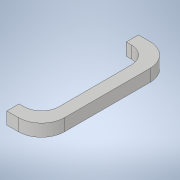
# Autodesk Inventor part: acc door handle
Saved by Autodesk Inventor 2020 (Build 240168000, 168)
## iProperties
Created: 2019-03-08
Part Number: acc door handle
Material: Generic
Document SubType Name: Modeling
Designer: aonih
Density: 1 g/cm^3
Appearance: Default
Author: aonih
Autodesk Inventor part; units mm, degrees
ref_plane "YZ Plane" through (0, 0, 0) normal (1, 0, 0) x (0, 1, 0)
ref_plane "XZ Plane" through (0, 0, 0) normal (0, 1, 0) x (-1, 0, 0)
ref_plane "XY Plane" through (0, 0, 0) normal (0, 0, 1) x (1, 0, 0)
sketch "Sketch1" plane through (0, 0, 0) normal (0, 1, 0) x (-1, 0, 0)
  line L0 (15, 57) -> (-15, 57)
  line L1 (-15, 57) -> (-15, -57)
  line L2 (-15, -57) -> (15, -57)
  line L3 (15, -57) -> (15, 57)
  line L4 (0, 57) -> (0, -57) construction
  line L5 (15, 0) -> (-15, 0) construction
  line L6 (15, 46.3934) -> (10.6066, 46.3934)
  line L7 (-4.3934, 31.3934) -> (-4.3934, -31.3934)
  line L8 (10.6066, -46.3934) -> (15, -46.3934)
  line L9 (15, -46.3934) -> (15, 46.3934)
  arc A0 (10.6066, 46.3934) -> (-4.3934, 31.3934) centre (10.6066, 31.3934) ccw
  arc A1 (-4.3934, -31.3934) -> (10.6066, -46.3934) centre (10.6066, -31.3934) ccw
  point P0 (0, 0)
  point P1 (-4.3934, -46.3934)
  point P2 (-4.3934, 46.3934)
  dimension "d0" = 114
  dimension "d1" = 30
  dimension "d4" = 15
  dimension "d5" = 10.6066
  dimension "d17" = 92.7868
  dimension "d20" = 15
  constraints: 20 end point, 7 midpoint, 4 parallel, 4 point on circle, 4 point on line, 4 tangent, 2 centre point, 2 horizontal, 2 perpendicular, 1 equal radius
  measures "d0" distance of L2.end L0.start
  measures "d1" distance of L1.end L2.end
  measures "d4" distance of L1.end point (-4.393, -46.393)
  measures "d5" distance between parallel lines of L1 L7
  measures "d17" distance between parallel lines of L8 L6
  measures "d20" radius of A0
extrude "Extrusion1" add sketch "Sketch1" along normal blind 10.6066 contours L3 L6 A0 L7 A1 L8 L2 L1 L0
sketch "Sketch4" plane through (4.3934, 0, 46.3934) normal (-1, 0, 0) x (0, 0, 1)
  circle A0 centre (5.2379, 5.2459) radius 2.1 projected
  circle A1 centre (-98.0247, 5.2459) radius 2.1 projected
  line L0 (5.2379, 5.2459) -> (-98.0247, 5.2459)
  point P0 (-46.3934, 0)
  dimension "d18" = 103.2627
  constraints: 2 end point, 1 horizontal
  measures "d18" distance of L0.start L0.end
fillet "Fillet2" radius 20 2 edges at (15, 5.3033, 57) (15, 5.3033, -57)
hole "Hole2" at (4.3934, 5.2459, 51.6313) direction (-1, 0, 0) diameter 4.2 end through all
mirror "Mirror2" about plane through (0, 0, 0) normal (0, 0, 1) of "Hole2"
equation "\"d6\" = d5"
body "Solid1"
